Autodesk Inventor part; units mm, degrees
(part 2 of 2)
  constraints: 1335 point on circle, 513 centre point, 8 end point, 6 coincident, 5 tangent, 2 equal radius, 2 vertical alignment, 1 point on line, 1 vertical, 1945 other
  measures "d33" radius of A10
extrude "Zahnprofil" cut sketch "Sketch3" against normal through all contours A1 A141 A137 A135 A134 | A136 A132 A130 A129 A1 | A1 A146 A142 A140 A139 | A131 A127 A125 A124 A1 | A1 A151 A147 A145 A144 | A126 A122 A120 A119 A1 | A1 A156 A152 A150 A149 | A121 A117 A115 A114 A1 | A1 A161 A157 A155 A154 | A116 A112 A110 A109 A1 | A1 A166 A162 A160 A159 | A111 A107 A105 A104 A1 | A1 A171 A167 A165 A164 | A106 A102 A100 A99 A1 | A1 A176 A172 A170 A169 | A101 A97 A95 A94 A1 | A1 A181 A177 A175 A174 | A96 A92 A90 A89 A1 | A1 A186 A182 A180 A179 | A91 A87 A85 A84 A1 | A1 A191 A187 A185 A184 | A86 A82 A80 A79 A1 | A1 A196 A192 A190 A189 | A81 A77 A75 A74 A1 | A1 A201 A197 A195 A194 | A76 A72 A70 A69 A1 | A1 A206 A202 A200 A199 | A71 A67 A65 A64 A1 | A1 A211 A207 A205 A204 | A66 A62 A60 A59 A1 | A1 A216 A212 A210 A209 | A61 A57 A55 A54 A1 | A1 A221 A217 A215 A214 | A56 A52 A50 A49 A1 | A1 A226 A222 A220 A219 | A51 A47 A45 A44 A1 | A1 A231 A227 A225 A224 | A46 A42 A40 A39 A1 | A1 A236 A232 A230 A229 | A41 A37 A35 A34 A1 | A1 A241 A237 A235 A234 | A36 A32 A30 A29 A1 | A1 A246 A242 A240 A239 | A31 A27 A25 A24 A1 | A1 A251 A247 A245 A244 | A26 A22 A20 A19 A1 | A1 A256 A252 A250 A249 | A21 A17 A15 A14 A1 | A1 A261 A257 A255 A254 | A16 A12 A4 A11 A1 | A1 A266 A262 A260 A259 | A10 A5 A515 A514 A1 | A1 A271 A267 A265 A264 | A516 A512 A510 A509 A1 | A1 A276 A272 A270 A269 | A511 A507 A505 A504 A1 | A1 A281 A277 A275 A274 | A506 A502 A500 A499 A1 | A1 A286 A282 A280 A279 | A501 A497 A495 A494 A1 | A1 A291 A287 A285 A284 | A496 A492 A490 A489 A1 | A1 A296 A292 A290 A289 | A491 A487 A485 A484 A1 | A1 A301 A297 A295 A294 | A486 A482 A480 A479 A1 | A1 A306 A302 A300 A299 | A481 A477 A475 A474 A1 | A1 A311 A307 A305 A304 | A476 A472 A470 A469 A1 | A1 A316 A312 A310 A309 | A471 A467 A465 A464 A1 | A1 A321 A317 A315 A314 | A466 A462 A460 A459 A1 | A1 A326 A322 A320 A319 | A461 A457 A455 A454 A1 | A1 A331 A327 A325 A324 | A456 A452 A450 A449 A1 | A1 A336 A332 A330 A329 | A451 A447 A445 A444 A1 | A1 A341 A337 A335 A334 | A446 A442 A440 A439 A1 | A1 A346 A342 A340 A339 | A441 A437 A435 A434 A1 | A1 A351 A347 A345 A344 | A436 A432 A430 A429 A1 | A1 A356 A352 A350 A349 | A431 A427 A425 A424 A1 | A1 A361 A357 A355 A354 | A426 A422 A420 A419 A1 | A1 A366 A362 A360 A359 | A421 A417 A415 A414 A1 | A1 A371 A367 A365 A364 | A416 A412 A410 A409 A1 | A1 A376 A372 A370 A369 | A411 A407 A405 A404 A1 | A1 A381 A377 A375 A374 | A406 A402 A400 A399 A1 | A1 A386 A382 A380 A379 | A401 A397 A395 A394 A1 | A1 A391 A387 A385 A384 | A396 A392 A390 A389 A1
sketch "Sketch4" plane through (0, 0, 10) normal (0, 0, 1) x (1, 0, 0)
  circle A0 centre (-40, 0) radius 3.925
  circle A1 centre (0, 0) radius 40 construction
  circle A2 centre (0, 0) radius 6.925 construction
  line L0 (-40, 0) -> (0, 0) construction
  circle A3 centre (0, 0) radius 40 construction
  circle A4 centre (0, -40) radius 3.925
  circle A5 centre (0, 0) radius 40 construction
  circle A6 centre (40, 0) radius 3.925
  circle A7 centre (0, 0) radius 40 construction
  circle A8 centre (0, 40) radius 3.925
  dimension "d42" = 80
  dimension "d40" = 7.85
  dimension "d45" = 360
  constraints: 4 centre point, 2 end point, 2 horizontal alignment, 2 vertical alignment, 1 coincident, 1 horizontal, 25 other
  measures "d40" diameter of A0
extrude "AdjustmentHoles" cut sketch "Sketch4" against normal through all
sketch "Sketch2" plane through (0, 0, 10) normal (0, 0, 1) x (1, 0, 0)
  line L0 (0, 17.5) -> (0, 0) construction
  circle A0 centre (0, 0) radius 17.5 construction
  point P0 (-15.1554, -8.75)
  point P1 (15.1554, -8.75)
  dimension "BigGear_Flansch" = 35
  dimension "d7" = 360
  constraints: 2 end point, 1 coincident, 1 vertical, 1 vertical alignment, 6 other
hole "Hole1" at (0, 17.5, 10) at (-15.1554, -8.75, 10) at (15.1554, -8.75, 10) direction (0, 0, -1) diameter 6.85 depth 11.8 tip angle 118
sketch "Sketch5" plane through (0, 0, 10) normal (0, 0, 1) x (1, 0, 0)
  circle A0 centre (0, 0) radius 6.925 projected
  circle A1 centre (0, 0) radius 80.599 construction
  arc A2 (0.3768, 80.5981) -> (-0.3768, 80.5981) centre (0, 0) ccw projected
  point P0 (0, 80.599)
  dimension "d49" = 161.198
  constraints: 1 coincident, 1 point on circle, 1 vertical alignment, 2 other
equation "\"Teilung\" = 5"
equation "\"GearDia\" = 162.33804"
equation "\"Dp_De_Diff_5\" = 1.14"
body "Solid1"
